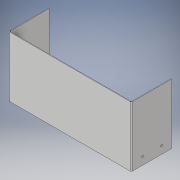
# Autodesk Inventor part: Chute
Saved by Autodesk Inventor 2017 (Build 210142000, 142)
## iProperties
Created: 2017-01-16
Part Number: Chute
Material: Generic
Document SubType Name: Sheet Metal
Designer: kingb
Density: 1 g/cm^3
Sheet Metal Rule: Default
Appearance: Default
Author: kingb
Autodesk Inventor part; units mm, degrees
ref_plane "YZ Plane" through (0, 0, 0) normal (1, 0, 0) x (0, 1, 0)
ref_plane "XZ Plane" through (0, 0, 0) normal (0, 1, 0) x (-1, 0, 0)
ref_plane "XY Plane" through (0, 0, 0) normal (0, 0, 1) x (1, 0, 0)
sketch "Sketch1" plane through (0, 0, 0) normal (0, 0, 1) x (1, 0, 0)
  line L0 (0, 0) -> (311.15, 0)
  line L1 (311.15, 0) -> (311.15, 152.4)
  line L2 (311.15, 152.4) -> (0, 152.4)
  line L3 (0, 152.4) -> (0, 0)
  dimension "d0" = 311.15
  dimension "d1" = 152.4
  measures "d0" distance of L2.end L1.end
  measures "d1" distance of L1.end L0.end
extrude "Plate1" add sketch "Sketch1" along normal blind 1.5875
sketch "Sketch2" plane through (309.5625, 0, 1.5875) normal (1, 0, 0) x (0, 1, 0)
  line L0 (152.4, 0) -> (0, 0)
  line L1 (0, 0) -> (0, -101.6)
  line L2 (0, -101.6) -> (152.4, -101.6)
  line L3 (152.4, -101.6) -> (152.4, 0)
  constraints: 6 end point, 1 horizontal, 1 perpendicular, 1 vertical
edge flange "Flange1" height 101.6 angle 90 thickness 1.5875 bend radius 1.5875 thickness toward (1, 0, 0) relief straight relief width 1.5875 relief depth 0.7937 corner gap 1.5875 corner form 0 edges at (311.15, 76.2, 0) (0, 76.2, 0) wall of the first edge with corners at (309.5625, 152.4, 1.5875) (309.5625, 0, 1.5875) (309.5625, 0, -100.0125) (309.5625, 152.4, -100.0125)
bend "Bend1"
corner "Corner1"
sketch "Sketch3" plane through (311.15, 0, -100.0125) normal (1, 0, 0) x (0, 0, -1)
  circle A0 centre (-73.025, 19.05) radius 2.54
  circle A1 centre (-25.4, 19.05) radius 2.54
  line L0 (0, 152.4) -> (0, 0) projected
  line L1 (-98.425, 152.4) -> (-98.425, 0) projected
  line L2 (0, 0) -> (-98.425, 0) projected
  point P0 (-100.0125, 0)
  dimension "d13" = 5.08
  dimension "d14" = 5.08
  dimension "d15" = 25.4
  dimension "d16" = 25.4
  dimension "d17" = 19.05
  dimension "d18" = 19.05
  constraints: 2 centre point
  measures "d13" diameter of A0
  measures "d14" diameter of A1
  measures "d15" distance from line of L0 A1.centre
  measures "d16" distance from line of L1 A0.centre
  measures "d17" distance from line of L2 A0.centre
  measures "d18" distance from line of L2 A1.centre
extrude "Extrusion1" cut sketch "Sketch3" against normal up to surface (311.15 mm away)
equation "\"d3\" = BendReliefWidth"
equation "\"d4\" = BendReliefDepth"
equation "\"d5\" = MinimumRemnant"
equation "\"d6\" = BendRadius"
equation "\"d9\" = BendRadius"
equation "\"d10\" = CornerReliefSize"
equation "\"d11\" = GapSize"
equation "\"d12\" = JacobiRadiusSize"
equation "\"BendRadius\" = Thickness"
equation "\"BendReliefWidth\" = Thickness"
equation "\"BendReliefDepth\" = 0.5 * Thickness"
equation "\"CornerReliefSize\" = 4 * Thickness"
equation "\"MinimumRemnant\" = 2 * Thickness"
equation "\"TransitionRadius\" = BendRadius"
equation "\"JacobiRadiusSize\" = Thickness"
equation "\"GapSize\" = Thickness"
equation "\"d2\" = BendRadius"
equation "\"Thickness\" = 1.5875"
body "Solid1"
